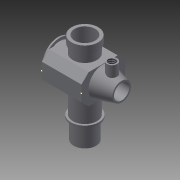
# Autodesk Inventor part: Carburetor Housing
Saved by Autodesk Inventor 2015 (Build 190159000, 159)
## iProperties
Created: 2016-02-13
Part Number: Carburetor Housing
Material: Generic
Document SubType Name: Modeling
Designer: Owner
Density: 1 g/cm^3
Appearance: Default
Author: Owner
Autodesk Inventor part; units mm, degrees
ref_plane "YZ Plane" through (0, 0, 0) normal (1, 0, 0) x (0, 1, 0)
ref_plane "XZ Plane" through (0, 0, 0) normal (0, 1, 0) x (-1, 0, 0)
ref_plane "XY Plane" through (0, 0, 0) normal (0, 0, 1) x (1, 0, 0)
sketch "Sketch1" plane through (0, 0, 0) normal (0, 1, 0) x (-1, 0, 0)
  line L0 (0, 0) -> (-17.5768, 0)
  line L1 (-17.5768, 0) -> (-17.5768, -19.2278)
  line L2 (-17.5768, -19.2278) -> (0, -19.2278)
  line L3 (0, -19.2278) -> (0, 0)
  dimension "d0" = 17.5768
  dimension "d1" = 19.2278
  constraints: 8 end point, 2 parallel, 1 horizontal, 1 perpendicular
  measures "d0" distance of L2.end L1.end
  measures "d1" distance of L1.end L0.end
extrude "Extrusion1" add sketch "Sketch1" along normal mid plane 13.1572
sketch "Sketch4" plane through (0, -6.5786, 0) normal (0, -1, 0) x (1, 0, 0)
  line L0 (17.5768, 0) -> (17.5768, -19.2278) projected
  circle A0 centre (9.4742, -9.6139) radius 5.3213
  point P0 (0, 0)
  dimension "d12" = 10.6426
  constraints: 1 centre point
  measures "d12" diameter of A0
extrude "Extrusion4" add sketch "Sketch4" along normal blind 10.2616
sketch "Sketch5" plane through (9.4742, -16.8402, -9.6139) normal (0, -1, 0) x (1, 0, 0)
  circle A0 centre (0, 0) radius 6.1595
  point P0 (-9.4742, 9.6139)
  dimension "d15" = 12.319
  constraints: 1 centre point
  measures "d15" diameter of A0
extrude "Extrusion5" add sketch "Sketch5" along normal blind 0.8382
sketch "Sketch2" plane through (0, 6.5786, 0) normal (0, 1, 0) x (1, 0, 0)
  line L0 (0, 19.2278) -> (0, 0) projected
  line L1 (17.5768, 19.2278) -> (0, 19.2278) projected
  line L2 (0, 0) -> (17.5768, 0) projected
  line L3 (17.5768, 0) -> (17.5768, 19.2278) projected
  line L4 (17.5768, 0) -> (9.4742, 0)
  circle A0 centre (9.4742, 9.6139) radius 5.3213
  dimension "d4" = 8.1026
  dimension "d5" = 10.6426
  constraints: 2 end point, 1 centre point, 1 point on line
  measures "d4" distance of L2.end L4.end
  measures "d5" diameter of A0
extrude "Extrusion2" add sketch "Sketch2" along normal blind 7.0612 contours A0
sketch "Sketch3" plane through (9.4742, 13.6398, -9.6139) normal (0, 1, 0) x (1, 0, 0)
  circle A0 centre (0, 0) radius 5.8674
  point P0 (-9.4742, -9.6139)
  dimension "d8" = 11.7348
  constraints: 1 centre point
  measures "d8" diameter of A0
extrude "Extrusion3" add sketch "Sketch3" against normal blind 3.2512
sketch "Sketch7" plane through (0, -6.5786, 0) normal (-1, 0, 0) x (0, 0, 1)
  line L0 (-19.2278, 13.1572) -> (0, 0) construction
  line L1 (-19.2278, 0) -> (-19.2278, 13.1572) projected
  line L2 (-19.2278, 6.5786) -> (-9.6139, 6.5786) construction
  circle A0 centre (-9.6139, 6.5786) radius 5.715
  point P0 (0, 6.5786)
  dimension "d21" = 11.43
  constraints: 4 end point, 2 midpoint, 1 centre point, 1 coincident
  measures "d21" diameter of A0
extrude "Extrusion7" add sketch "Sketch7" along normal blind 2.286
sketch "Sketch8" plane through (-2.286, 0, -9.6139) normal (-1, 0, 0) x (0, 0, 1)
  circle A0 centre (0, 0) radius 6.9596
  point P0 (9.6139, 0)
  dimension "d24" = 13.9192
  constraints: 1 centre point
  measures "d24" diameter of A0
extrude "Extrusion8" add sketch "Sketch8" against normal blind 0.6858
sketch "Sketch6" plane through (9.4742, -17.6784, -9.6139) normal (0, -1, 0) x (1, 0, 0)
  circle A0 centre (0, 0) radius 4.953
  point P0 (-9.4742, 9.6139)
  dimension "d18" = 9.906
  constraints: 1 centre point
  measures "d18" diameter of A0
extrude "Extrusion6" add sketch "Sketch6" along normal blind 8.763
sketch "Sketch9" plane through (0, 0, 0) normal (0, 0, 1) x (1, 0, 0)
  point P0 (0, 0)
ref_plane "Work Plane1" through (0, 6.5786, -9.6139) normal (0, 0, 1) x (1, 0, 0)
sketch "Sketch11" plane through (0, 0, 0) normal (0, 1, 0) x (-1, 0, 0)
  line L0 (-25.7556, -5.4737) -> (-25.7556, -13.7541) projected
  line L1 (-25.7556, -9.6139) -> (-21.4884, -9.6139)
  circle A0 centre (-21.4884, -9.6139) radius 2.2225
  point P0 (0, 0)
  dimension "d31" = 4.2672
  dimension "d32" = 4.445
  constraints: 2 end point, 1 centre point, 1 coincident, 1 horizontal, 1 midpoint
  measures "d31" distance of L1.start L1.end
  measures "d32" diameter of A0
extrude "Extrusion9" add sketch "Sketch11" along normal blind 9.525
ref_plane "Work Plane3" through (25.7556, -6.5786, -19.2278) normal (1, 0, 0) x (0, 0, -1)
sketch "Sketch12" plane through (17.5768, -6.5786, -19.2278) normal (1, 0, 0) x (0, 0, -1)
  point P0 (-19.2278, 6.5786)
sketch "Sketch13" plane through (17.5768, -6.5786, -19.2278) normal (1, 0, 0) x (0, 0, -1)
  circle A0 centre (-9.7674, 6.5786) radius 6.4008
  point P0 (-19.2278, 6.5786)
  dimension "d36" = 12.8016
  constraints: 1 centre point
  measures "d36" diameter of A0
sketch "Sketch14" plane through (25.7556, -6.5786, -19.2278) normal (1, 0, 0) x (0, 0, -1)
  line L0 (-11.8364, 6.5786) -> (-7.3914, 6.5786) projected
  circle A0 centre (-9.6139, 6.5786) radius 4.1402
  point P0 (-19.2278, 6.5786)
  dimension "d37" = 8.2804
  constraints: 1 centre point, 1 midpoint
  measures "d37" diameter of A0
loft "Loft1" add profiles "Sketch13", "Sketch14"
chamfer "Chamfer1" distance 3.175 angle 45 4 edges at (8.7884, 6.5786, -19.2278) (8.7884, -6.5786, -19.2278) (8.7884, -6.5786, 0) (8.7884, 6.5786, 0)
hole "Hole1" at (-2.286, 0, -9.6139) direction (1, 0, 0) diameter 10.5918 depth 16.8402
hole "Hole2" at (9.4742, 13.6398, -9.6139) direction (0, -1, 0) diameter 9.0678 end through all
hole "Hole3" at (25.7556, 0, -9.6139) direction (-1, 0, 0) diameter 6.8072 end through all
hole "Hole4" at (21.4884, 9.525, -9.6139) direction (0, -1, 0) diameter 3.302 depth 10.16 tip angle 118 thread size "8-32 UNC" class "2B" standard "ANSI Unified Screw Threads"
body "Solid1"
